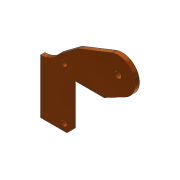
# Autodesk Inventor part: HIP_TOPFRAME2
Saved by Autodesk Inventor 2019.4 (Build 234330000, 330)
## iProperties
Created: 2019-11-06
Part Number: HIP_TOPFRAME2
Material: 一般
Document SubType Name: Modeling
Designer: y6tada
Density: 1 g/cm^3
Appearance: 滑らか - 淡いオレンジ
Author: y6tada
Autodesk Inventor part; units mm, degrees
ref_plane "YZ Plane" through (0, 0, 0) normal (1, 0, 0) x (0, 1, 0)
ref_plane "XZ Plane" through (0, 0, 0) normal (0, 1, 0) x (-1, 0, 0)
ref_plane "XY Plane" through (0, 0, 0) normal (0, 0, 1) x (1, 0, 0)
sketch "スケッチ1" plane through (0, 0, 0) normal (0, 0, 1) x (0, 1, 0)
  circle A0 centre (12, 0) radius 4 construction
  arc A1 (2, 0) -> (6.1183, -8.0874) centre (12, 0) ccw
  arc A2 (6.8885, -8.8489) -> (6.1183, -8.0874) centre (4, -11) ccw
  line L0 (-23.25, 12.25) -> (-23.25, -12.25) construction
  line L1 (-23.25, -12.25) -> (-21.25, -14.25) construction
  line L2 (-21.25, -14.25) -> (21.25, -14.25) construction
  line L3 (0, 0) -> (2, 0)
  line L4 (0, 0) -> (-23.25, 0)
  line L5 (-23.25, 0) -> (-23.25, -12.25)
  line L6 (-23.25, -12.25) -> (-21.25, -14.25)
  line L7 (-0.4772, -29.5258) -> (4.929, -39.7419)
  line L8 (6.8885, -8.8489) -> (13.2614, -17.4062)
  line L9 (13.2614, -17.4062) -> (19.4413, -33.0628)
  line L10 (2, 0) -> (12, 0) construction
  circle A3 centre (4, -11) radius 1.25 construction
  arc A4 (4.929, -39.7419) -> (19.4413, -33.0628) centre (12, -36) ccw
  circle A5 centre (-20, -11) radius 1.25 construction
  line L11 (12, 0) -> (12, -36) construction
  line L12 (-21.25, -14.25) -> (-0.4772, -14.25)
  line L13 (-0.4772, -29.5258) -> (-0.4772, -14.25)
  dimension "d0" = 10
  dimension "d3" = 36
  dimension "d4" = 8
  constraints: 22 end point, 6 point on circle, 4 tangent, 3 centre point, 3 coincident, 2 collinear, 2 concentric, 2 horizontal, 1 midpoint, 1 point on line, 1 vertical
  measures "d0" radius of A1
  measures "d3" distance of L11.start L11.end
  measures "d4" radius of A4
extrude "押し出し1" add sketch "スケッチ1" along normal blind 2
hole "穴1" at (36, 12, 0) direction (0, 0, 1) diameter 3 end through all
hole "穴2" at (11, 4, 0) at (11, -20, 0) direction (0, 0, 1) diameter 2.5 end through all
